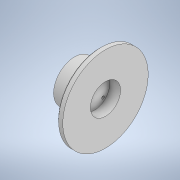
# Autodesk Inventor part: Gegestuck
Saved by Autodesk Inventor 2021 (Build 250183000, 183)
## iProperties
Created: 2024-02-01
Part Number: Gegestuck
Material: Generic
Document SubType Name: Modeling
Designer: Lukas
Density: 1 g/cm^3
Appearance: Default
Author: Lukas
Autodesk Inventor part; units mm, degrees
ref_plane "YZ Plane" through (0, 0, 0) normal (1, 0, 0) x (0, 1, 0)
ref_plane "XZ Plane" through (0, 0, 0) normal (0, 1, 0) x (-1, 0, 0)
sketch "Sketch1" plane through (0, 0, 0) normal (0, 0, 1) x (1, 0, 0)
  line L0 (0, 0) -> (0, 25)
  line L1 (0, 25) -> (32, 25)
  line L2 (32, 25) -> (32, 43)
  line L3 (32, 43) -> (30, 45)
  line L4 (30, 45) -> (30, 49)
  line L5 (30, 49) -> (32, 51)
  line L6 (32, 51) -> (37, 51)
  line L7 (24, 0) -> (0, 0)
  line L8 (37, 51) -> (37, 18)
  line L9 (37, 18) -> (24, 18)
  line L10 (24, 18) -> (24, 0)
  line L11 (-7.4, 0) -> (44.4, 0) projected
  dimension "d0" = 25
  dimension "d1" = 30
  dimension "d2" = 2
  dimension "d3" = 2
  dimension "d4" = 2
  dimension "d5" = 4
  dimension "d6" = 5
  dimension "d7" = 45
  dimension "d8" = 18
  dimension "d9" = 24
  constraints: 23 end point, 4 perpendicular, 2 parallel, 2 vertical, 1 point on line
  measures "d0" distance between parallel lines of L7 L1
  measures "d1" distance between parallel lines of L4 L0
  measures "d2" horizontal distance of L4.end L5.end
  measures "d3" horizontal distance of L4.end L5.end
  measures "d4" horizontal distance of L2.end L3.end
  measures "d5" distance of L3.end L4.end
  measures "d6" distance of L5.end L6.end
  measures "d7" vertical distance of L0.start L3.end
  measures "d8" distance from line of L0.start L9
  measures "d9" distance between parallel lines of L0 L10
revolve "Revolution1" add sketch "Sketch1" angle 360 about axis through (-10, 0, 0) along (1, 0, 0)
ref_plane "Work Plane1" through (0, 0, 30) normal (0, 0, 1) x (1, 0, 0)
sketch "Sketch2" plane through (0, 0, 30) normal (0, 0, 1) x (1, 0, 0)
  line L0 (30, -49) -> (30, 49) projected
  line L1 (30, 2.5) -> (31, 1.5)
  line L2 (31, 1.5) -> (31, -1.5)
  line L3 (32, -25) -> (32, 25) projected
  line L4 (31, -1.5) -> (30, -2.5)
  point P0 (0, 0)
  point P1 (31, 0)
  dimension "d12" = 3
  dimension "d13" = 1
  dimension "d14" = 1
  dimension "d15" = 1
  constraints: 6 end point, 2 point on line, 1 horizontal alignment, 1 midpoint, 1 parallel
  measures "d12" distance of L1.end L2.end
  measures "d13" distance between parallel lines of L0 L2
  measures "d14" horizontal distance of L1.start L1.end
  measures "d15" horizontal distance of L2.end L4.end
extrude "Extrusion1" cut sketch "Sketch2" along normal through all
pattern_circular "Circular Pattern1" count 36 over 360 about axis through (-10, 0, 0) along (1, 0, 0) of "Extrusion1"
sketch "Sketch3" plane through (0, 0, 0) normal (-1, 0, 0) x (0, 0, 1)
  circle A0 centre (-10, 10) radius 1.6
  circle A1 centre (10, 10) radius 1.6
  circle A2 centre (10, -10) radius 1.6
  circle A3 centre (-10, -10) radius 1.6
  point P0 (0, 0)
  dimension "d21" = 20
  dimension "d22" = 20
  dimension "d23" = 10
  dimension "d24" = 10
  dimension "d25" = 3.2
  constraints: 4 centre point, 3 equal radius, 2 horizontal alignment, 2 vertical alignment
  measures "d21" distance of A1.centre A0.centre
  measures "d22" distance of A2.centre A1.centre
  measures "d23" horizontal distance of point (0, 0) A0.centre
  measures "d24" horizontal distance of point (0, 0) A1.centre
  measures "d25" diameter of A0
extrude "Extrusion2" cut sketch "Sketch3" against normal through all
equation "\"d4\" = d3"
equation "\"d15\" = d14"
equation "\"d22\" = d21"
equation "\"d23\" = 0.5 * d21"
equation "\"d24\" = 0.5 * d22"
body "Solid1"
